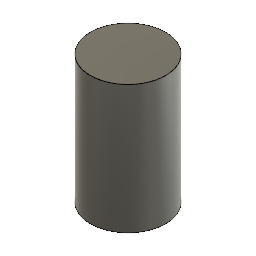
DisplayEnclosure_ButtonSpacer_v2 (Autodesk Fusion 360 design; units mm, degrees)
Autodesk Fusion 360 part; units mm, degrees
sketch "Sketch1" plane through (0, 0, 0) normal (0, 1, 0) x (1, 0, 0)
  circle A0 centre (0, 0) radius 1.7
  dimension "d1" = 3.4
  constraint coincident A0.centre origin
  measures "d1" diameter of A0
extrude "Extrude1" add sketch "Sketch1" along normal blind 6
extrude "Extrude2" cut 1 faces at (-0.3785, 6, -0.6303) along direction (0, -1, 0) blind 0.2
